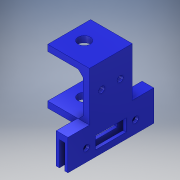
# Autodesk Inventor part: Suspension Frame 3.0
Saved by Autodesk Inventor 2018.2 (Build 222227000, 227)
## iProperties
Created: 2018-03-16
Part Number: Suspension Frame 3.0
Material: Generic
Document SubType Name: Modeling
Designer: MIABo
Density: 1 g/cm^3
Appearance: Default
Author: MIABo
## iProperties of the stored document Suspension Frame 3_3DPrint.ipt
Created: 2018-03-16
Part Number: Suspension Frame 3_3DPrint
Material: Generic
Document SubType Name: Modeling
Designer: MIABo
Density: 1 g/cm^3
Appearance: Default
Author: MIABo
Autodesk Inventor part; units mm, degrees
ref_plane "YZ Plane" through (0, 0, 0) normal (1, 0, 0) x (0, 1, 0)
ref_plane "XZ Plane" through (0, 0, 0) normal (0, 1, 0) x (-1, 0, 0)
ref_plane "XY Plane" through (0, 0, 0) normal (0, 0, 1) x (1, 0, 0)
sketch "Sketch1" plane through (0, 0, 0) normal (0, 0, 1) x (1, 0, 0)
  line L0 (-2.8575, 0) -> (-2.8575, -25.4)
  line L1 (-2.8575, -25.4) -> (-6.0325, -25.4)
  line L2 (-6.0325, -25.4) -> (-6.0325, 6.35)
  line L3 (2.8575, 0) -> (2.8575, -25.4)
  line L4 (2.8575, -25.4) -> (6.0325, -25.4)
  line L5 (6.0325, -25.4) -> (6.0325, 6.35)
  line L6 (-6.0325, 6.35) -> (6.0325, 6.35)
  line L7 (2.8575, 0) -> (-2.8575, 0)
  point P0 (0, 0)
  point P1 (0, 0)
  dimension "d0" = 5.715
  dimension "d1" = 3.175
  dimension "d2" = 25.4
  dimension "d3" = 31.75
  constraints: 16 end point, 3 perpendicular, 2 horizontal, 2 point on line, 1 coincident, 1 collinear, 1 midpoint, 1 vertical, 1 other
  measures "d0" distance between parallel lines of L3 L0
  measures "d1" distance of L0.end L1.end
  measures "d2" distance of L0.start L0.end
  measures "d3" distance of L4.end L5.end
extrude "Extrusion1" add sketch "Sketch1" along normal blind 88.9
sketch "Sketch2" plane through (-6.0325, -25.4, 0) normal (-1, 0, 0) x (0, 0, 1)
  line L0 (22.225, 31.75) -> (66.675, 31.75)
  line L1 (66.675, 31.75) -> (66.675, 25.4)
  line L2 (66.675, 25.4) -> (22.225, 25.4)
  line L3 (22.225, 25.4) -> (22.225, 31.75)
  line L4 (0, 31.75) -> (88.9, 31.75) projected
  point P0 (0, 25.4)
  point P1 (44.45, 31.75)
  dimension "d9" = 6.35
  dimension "d10" = 44.45
  constraints: 8 end point, 2 midpoint, 2 parallel, 1 collinear, 1 horizontal, 1 perpendicular
  measures "d9" distance of L2.end L0.start
  measures "d10" distance of L1.end L2.end
extrude "Extrusion2" add sketch "Sketch2" along normal blind 31.115
sketch "Sketch3" plane through (-6.0325, 6.35, 0) normal (0, 1, 0) x (1, 0, 0)
  line L0 (12.065, 0) -> (12.065, -88.9) projected
  line L1 (12.065, -22.225) -> (5.715, -22.225)
  line L2 (5.715, -22.225) -> (5.715, -66.675)
  line L3 (5.715, -66.675) -> (12.065, -66.675)
  line L4 (12.065, -66.675) -> (12.065, -22.225)
  line L5 (0, -22.225) -> (-31.115, -22.225) projected
  line L6 (0, -66.675) -> (-31.115, -66.675) projected
  point P0 (6.0325, 0)
  dimension "d13" = 6.35
  constraints: 8 end point, 2 collinear, 2 parallel, 1 horizontal, 1 perpendicular, 1 point on line
  measures "d13" distance of L1.start L1.end
extrude "Extrusion3" add sketch "Sketch3" along normal blind 50.8
sketch "Sketch4" plane through (-0.3175, 57.15, 22.225) normal (-1, 0, 0) x (0, 0, 1)
  line L0 (0, -50.8) -> (0, 0) projected
  line L1 (44.45, 0) -> (0, 0)
  line L2 (0, 0) -> (0, -6.35)
  line L3 (0, -6.35) -> (44.45, -6.35)
  line L4 (44.45, -6.35) -> (44.45, 0)
  line L5 (0, 0) -> (44.45, 0) projected
  line L6 (44.45, -50.8) -> (44.45, 0) projected
  point P0 (-22.225, -57.15)
  point P1 (44.45, -45.72)
  dimension "d17" = 6.35
  constraints: 8 end point, 2 collinear, 2 parallel, 1 horizontal, 1 perpendicular, 1 point on line
  measures "d17" distance of L3.end L1.start
extrude "Extrusion4" add sketch "Sketch4" along normal up to surface (36.83 mm away)
chamfer "Chamfer1" distance 5.08 angle 45 1 edges at (-0.3175, 50.8, 44.45)
chamfer "Chamfer2" distance 5.08 angle 45 1 edges at (-0.3175, 6.35, 44.45)
chamfer "Chamfer3" distance 5.08 angle 45 1 edges at (-6.0325, 0, 44.45)
sketch "Sketch5" plane through (6.0325, -25.4, 0) normal (1, 0, 0) x (0, 0, -1)
  line L0 (-88.9, 0) -> (-88.9, 31.75) projected
  line L1 (0, 31.75) -> (0, 0) projected
  line L2 (0, 0) -> (-88.9, 0) projected
  point P0 (0, 25.4)
  point P1 (-69.85, 12.7)
  point P2 (-19.05, 12.7)
  dimension "d29" = 19.05
  dimension "d30" = 19.05
  dimension "d31" = 12.7
  dimension "d32" = 12.7
  measures "d29" distance from line of L0 point (-69.85, 12.7)
  measures "d30" distance from line of L1 point (-19.05, 12.7)
  measures "d31" distance from line of L2 point (-69.85, 12.7)
  measures "d32" distance from line of L2 point (-19.05, 12.7)
hole "Hole1" at (6.0325, -12.7, 69.85) at (6.0325, -12.7, 19.05) direction (-1, 0, 0) diameter 6.35 end through all
sketch "Sketch6" plane through (6.0325, -25.4, 0) normal (1, 0, 0) x (0, 0, -1)
  line L0 (-28.575, 6.35) -> (-60.325, 6.35)
  line L1 (-60.325, 6.35) -> (-60.325, 19.05)
  line L2 (-60.325, 19.05) -> (-28.575, 19.05)
  line L3 (-28.575, 19.05) -> (-28.575, 6.35)
  circle A0 centre (-69.85, 12.7) radius 3.175 projected
  circle A1 centre (-19.05, 12.7) radius 3.175 projected
  line L4 (0, 0) -> (-88.9, 0) projected
  point P0 (0, 25.4)
  dimension "d40" = 31.75
  dimension "d41" = 50.8
  dimension "d42" = 9.525
  dimension "d43" = 12.7
  dimension "d44" = 6.35
  constraints: 8 end point, 2 parallel, 1 horizontal, 1 perpendicular
  measures "d40" distance between parallel lines of L1 L3
  measures "d41" distance of A0.centre A1.centre
  measures "d42" distance from line of L1 A0.centre
  measures "d43" distance of L2.end L0.start
  measures "d44" distance between parallel lines of L4 L0
extrude "Extrusion5" cut sketch "Sketch6" against normal blind 50.8 contours L0 L1 L2 L3
sketch "Sketch7" plane through (-6.0325, 57.15, 0) normal (0, 1, 0) x (1, 0, 0)
  circle A0 centre (-15.5575, -44.45) radius 6.35
  line L0 (-31.115, -22.225) -> (-31.115, -66.675) projected
  line L1 (0, -22.225) -> (0, -66.675) projected
  line L2 (12.065, -66.675) -> (-31.115, -66.675) projected
  line L3 (12.065, -22.225) -> (-31.115, -22.225) projected
  point P0 (6.0325, 0)
  dimension "d47" = 15.5575
  dimension "d48" = 31.115
  dimension "d49" = 44.45
  dimension "d50" = 22.225
  dimension "d51" = 12.7
  constraints: 1 centre point
  measures "d47" distance from line of L0 A0.centre
  measures "d48" distance between parallel lines of L0 L1
  measures "d49" distance between parallel lines of L2 L3
  measures "d50" distance from line of L2 A0.centre
  measures "d51" diameter of A0
extrude "Extrusion6" cut sketch "Sketch7" against normal blind 101.6 contours A0
sketch "Sketch8" plane through (6.0325, -25.4, 0) normal (1, 0, 0) x (0, 0, -1)
  line L0 (-66.675, 31.75) -> (-66.675, 82.55) projected
  line L1 (-66.675, 82.55) -> (-22.225, 82.55) projected
  point P0 (0, 25.4)
  point P1 (-53.975, 57.15)
  point P2 (-34.925, 57.15)
  dimension "d54" = 19.05
  dimension "d55" = 12.7
  dimension "d56" = 25.4
  dimension "d57" = 50.8
  dimension "d58" = 25.4
  measures "d54" distance of point (-34.925, 57.15) point (-53.975, 57.15)
  measures "d55" distance from line of L0 point (-53.975, 57.15)
  measures "d56" distance from line of L1 point (-53.975, 57.15)
  measures "d57" distance of L0.start L0.end
  measures "d58" distance from line of L1 point (-34.925, 57.15)
hole "Hole2" at (6.0325, 31.75, 53.975) at (6.0325, 31.75, 34.925) direction (-1, 0, 0) diameter 6.35 end through all
equation "\"d47\" = 0.5 * d48"
equation "\"d50\" = 0.5 * d49"
equation "\"d56\" = 0.5 * d57"
body "Solid1"
